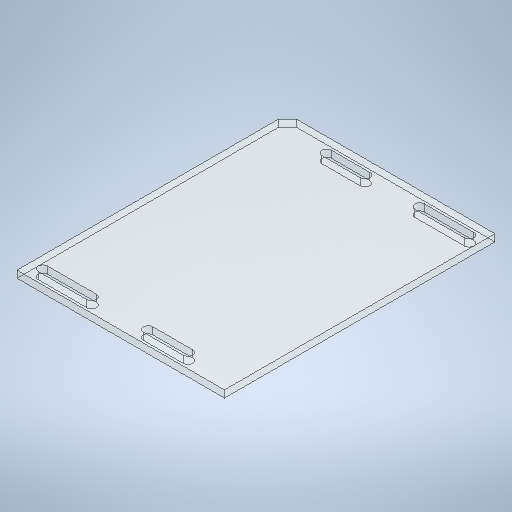
# Autodesk Inventor part: Flex Holder V1 TPMockup
Saved by Autodesk Inventor 2025 (Build 290162000, 162)
## iProperties
Created: 2025-07-01
Part Number: Flex Holder V1 TPMockup
Material: Thermoplastic Resin
Document SubType Name: Modeling
Designer: Caleb Fangmeier
Density: 1.28 g/cm^3
Appearance: Clear
Author: Caleb Fangmeier
Autodesk Inventor part; units mm, degrees
ref_plane "YZ Plane" through (0, 0, 0) normal (1, 0, 0) x (0, 1, 0)
ref_plane "XZ Plane" through (0, 0, 0) normal (0, 1, 0) x (-1, 0, 0)
ref_plane "XY Plane" through (0, 0, 0) normal (0, 0, 1) x (1, 0, 0)
sketch "Sketch1" plane through (0, 0, 0) normal (0, 1, 0) x (-1, 0, 0)
  line L0 (-22.05, -28.75) -> (22.05, -28.75)
  line L1 (22.05, -28.75) -> (22.05, 28.75)
  line L2 (22.05, 28.75) -> (-22.05, 28.75)
  line L3 (-22.05, 28.75) -> (-22.05, -28.75)
  line L4 (-22.05, -28.75) -> (22.05, 28.75) construction
  line L5 (22.05, -28.75) -> (-22.05, 28.75) construction
  point P0 (0, 0)
  dimension "d0" = 57.5
  dimension "d1" = 44.1
  constraints: 12 end point, 2 midpoint, 2 parallel, 1 horizontal, 1 perpendicular
  measures "d0" distance of L0.end L1.end
  measures "d1" distance of L1.end L2.end
extrude "Extrusion1" add sketch "Sketch1" along normal blind 1.5
sketch "Sketch4" plane through (0, 1.5, 0) normal (0, 1, 0) x (1, 0, 0)
  line L0 (22.6381, -25.9185) -> (13.7388, -25.9185)
  line L1 (13.7388, -25.9185) -> (13.7388, -21.956)
  line L2 (13.7388, -21.956) -> (22.6381, -21.956)
  line L3 (22.6381, -21.956) -> (22.6381, -25.9185)
  line L4 (11.4165, -21.956) -> (0.7633, -21.956)
  line L5 (0.7633, -21.956) -> (0.7633, -24.4569)
  line L6 (0.7633, -24.4569) -> (11.4165, -24.4569)
  line L7 (11.4165, -24.4569) -> (11.4165, -21.956)
  line L8 (-0.6658, -26.6006) -> (-6.707, -26.6006)
  line L9 (-6.707, -26.6006) -> (-6.707, -22.3783)
  line L10 (-6.707, -22.3783) -> (-0.6658, -22.3783)
  line L11 (-0.6658, -22.3783) -> (-0.6658, -26.6006)
  line L12 (-6.707, -24.392) -> (-14.5426, -24.392)
  line L13 (-14.5426, -24.392) -> (-14.5426, -21.0953)
  line L14 (-14.5426, -21.0953) -> (-6.707, -21.0953)
  line L15 (-6.707, -21.0953) -> (-6.707, -24.392)
  line L16 (-14.5426, -21.0953) -> (-11.8996, -21.0953)
  line L17 (-11.8996, -21.0953) -> (-11.8996, -19.5363)
  line L18 (-11.8996, -19.5363) -> (-14.5426, -19.5363)
  line L19 (-14.5426, -19.5363) -> (-14.5426, -21.0953)
  line L20 (-21.1238, -24.2621) -> (-17.4211, -24.2621)
  line L21 (-17.4211, -24.2621) -> (-17.4211, -21.956)
  line L22 (-17.4211, -21.956) -> (-21.1238, -21.956)
  line L23 (-21.1238, -21.956) -> (-21.1238, -24.2621)
  line L24 (5.6616, -20.7705) -> (1.894, -20.7705)
  line L25 (1.894, -20.7705) -> (1.894, -17.3277)
  line L26 (1.894, -17.3277) -> (5.6616, -17.3277)
  line L27 (5.6616, -17.3277) -> (5.6616, -20.7705)
  line L28 (-2.848, -19.9261) -> (-5.2515, -19.9261)
  line L29 (-5.2515, -19.9261) -> (-5.2515, -18.3346)
  line L30 (-5.2515, -18.3346) -> (-2.848, -18.3346)
  line L31 (-2.848, -18.3346) -> (-2.848, -19.9261)
  line L32 (-17.2689, -17.0029) -> (-14.5426, -17.0029)
  line L33 (-14.5426, -17.0029) -> (-14.5426, -13.4952)
  line L34 (-14.5426, -13.4952) -> (-17.2689, -13.4952)
  line L35 (-17.2689, -13.4952) -> (-17.2689, -17.0029)
  line L36 (15.925, -11.4814) -> (12.4173, -11.4814)
  line L37 (12.4173, -11.4814) -> (12.4173, -14.7294)
  line L38 (12.4173, -14.7294) -> (15.925, -14.7294)
  line L39 (15.925, -14.7294) -> (15.925, -11.4814)
  line L40 (-2.1335, 9.0455) -> (1.894, 9.0455)
  line L41 (1.894, 9.0455) -> (1.894, -8.9481)
  line L42 (1.894, -8.9481) -> (-2.1335, -8.9481)
  line L43 (-2.1335, -8.9481) -> (-2.1335, 9.0455)
  line L44 (4.5573, 3.3291) -> (1.6991, 3.3291)
  line L45 (1.6991, 3.3291) -> (1.6991, 0.6009)
  line L46 (1.6991, 0.6009) -> (4.5573, 0.6009)
  line L47 (4.5573, 0.6009) -> (4.5573, 3.3291)
  line L48 (-17.5287, 13.7631) -> (-14.1519, 13.7631)
  line L49 (-14.1519, 13.7631) -> (-14.1519, 10.4096)
  line L50 (-14.1519, 10.4096) -> (-17.5287, 10.4096)
  line L51 (-17.5287, 10.4096) -> (-17.5287, 13.7631)
  line L52 (16.8052, 16.3739) -> (14.7212, 16.3739)
  line L53 (14.7212, 16.3739) -> (14.7212, 12.9633)
  line L54 (14.7212, 12.9633) -> (16.8052, 12.9633)
  line L55 (16.8052, 12.9633) -> (16.8052, 16.3739)
  line L56 (-23.3919, 26.0219) -> (-13.2211, 26.0219)
  line L57 (-13.2211, 26.0219) -> (-13.2211, 21.0711)
  line L58 (-13.2211, 21.0711) -> (-23.3919, 21.0711)
  line L59 (-23.3919, 21.0711) -> (-23.3919, 26.0219)
  line L60 (-20.3793, 16.7032) -> (-17.8455, 16.7032)
  line L61 (-17.8455, 16.7032) -> (-17.8455, 19.4346)
  line L62 (-17.8455, 19.4346) -> (-20.3793, 19.4346)
  line L63 (-20.3793, 19.4346) -> (-20.3793, 16.7032)
  line L64 (-11.1745, 21.8169) -> (-0.7032, 21.8169)
  line L65 (-0.7032, 21.8169) -> (-0.7032, 24.5446)
  line L66 (-0.7032, 24.5446) -> (-11.1745, 24.5446)
  line L67 (-11.1745, 24.5446) -> (-11.1745, 21.8169)
  line L68 (-2.5673, 18.6812) -> (-4.8458, 18.6812)
  line L69 (-4.8458, 18.6812) -> (-4.8458, 22.2038)
  line L70 (-4.8458, 22.2038) -> (-2.5673, 22.2038)
  line L71 (-2.5673, 22.2038) -> (-2.5673, 18.6812)
  line L72 (0.9146, 27.1153) -> (6.539, 27.1153)
  line L73 (6.539, 27.1153) -> (6.539, 22.2038)
  line L74 (6.539, 22.2038) -> (0.9146, 22.2038)
  line L75 (0.9146, 22.2038) -> (0.9146, 27.1153)
  line L76 (2.2307, 17.9158) -> (4.5573, 17.9158)
  line L77 (4.5573, 17.9158) -> (4.5573, 22.2038)
  line L78 (4.5573, 22.2038) -> (2.2307, 22.2038)
  line L79 (2.2307, 22.2038) -> (2.2307, 17.9158)
  line L80 (6.0899, 24.1958) -> (14.5454, 24.1958)
  line L81 (14.5454, 24.1958) -> (14.5454, 21.5323)
  line L82 (14.5454, 21.5323) -> (6.0899, 21.5323)
  line L83 (6.0899, 21.5323) -> (6.0899, 24.1958)
  line L84 (14.2886, 21.5323) -> (11.9019, 21.5323)
  line L85 (11.9019, 21.5323) -> (11.9019, 19.3557)
  line L86 (11.9019, 19.3557) -> (14.2886, 19.3557)
  line L87 (14.2886, 19.3557) -> (14.2886, 21.5323)
  line L88 (21.4363, 24.0758) -> (17.64, 24.0758)
  line L89 (17.64, 24.0758) -> (17.64, 21.5323)
  line L90 (17.64, 21.5323) -> (21.4363, 21.5323)
  line L91 (21.4363, 21.5323) -> (21.4363, 24.0758)
  point P0 (0, 0)
  point P1 (6.539, 24.1958)
  point P2 (6.0899, 22.2038)
  constraints: 184 end point, 46 parallel, 23 perpendicular, 22 horizontal, 3 point on line
extrude "Clearance Cutouts" [suppressed]
sketch "Sketch5" plane through (0, 1.5, 0) normal (0, 1, 0) x (1, 0, 0)
  line L0 (19.55, 25.75) -> (9.039, 25.75) construction
  line L1 (19.55, 26.75) -> (9.039, 26.75)
  line L2 (9.039, 24.75) -> (19.55, 24.75)
  arc A0 (19.55, 24.75) -> (19.55, 26.75) centre (19.55, 25.75) ccw
  arc A1 (9.039, 26.75) -> (9.039, 24.75) centre (9.039, 25.75) ccw
  line L3 (22.05, -28.75) -> (22.05, 28.75) projected
  line L4 (-2.5854, 25.75) -> (-10.7211, 25.75) construction
  line L5 (-2.5854, 24.75) -> (-10.7211, 24.75)
  line L6 (-10.7211, 26.75) -> (-2.5854, 26.75)
  arc A2 (-2.5854, 24.75) -> (-2.5854, 26.75) centre (-2.5854, 25.75) ccw
  arc A3 (-10.7211, 26.75) -> (-10.7211, 24.75) centre (-10.7211, 25.75) ccw
  line L7 (-19.55, -25.75) -> (-9.207, -25.75) construction
  line L8 (-22.05, -28.75) -> (22.05, -28.75) projected
  line L9 (-19.55, -26.75) -> (-9.207, -26.75)
  line L10 (-9.207, -24.75) -> (-19.55, -24.75)
  arc A4 (-19.55, -24.75) -> (-19.55, -26.75) centre (-19.55, -25.75) ccw
  arc A5 (-9.207, -26.75) -> (-9.207, -24.75) centre (-9.207, -25.75) ccw
  line L11 (-22.05, 28.75) -> (-22.05, -28.75) projected
  line L12 (2.8342, -25.75) -> (11.2388, -25.75) construction
  line L13 (2.8342, -26.75) -> (11.2388, -26.75)
  line L14 (11.2388, -24.75) -> (2.8342, -24.75)
  arc A6 (2.8342, -24.75) -> (2.8342, -26.75) centre (2.8342, -25.75) ccw
  arc A7 (11.2388, -26.75) -> (11.2388, -24.75) centre (11.2388, -25.75) ccw
  line L15 (22.05, 28.75) -> (-22.05, 28.75) projected
  point P0 (0, 0)
  point P1 (14.2945, 25.75)
  point P2 (8.039, 25.75)
  point P3 (20.55, 25.75)
  point P4 (-6.6533, 25.75)
  point P5 (-1.5854, 25.75)
  point P6 (-11.7211, 25.75)
  point P7 (-14.3785, -25.75)
  point P8 (-8.207, -25.75)
  point P9 (-20.55, -25.75)
  point P10 (7.0365, -25.75)
  point P11 (1.8342, -25.75)
  point P12 (12.2388, -25.75)
  dimension "d23" = 2
  dimension "d26" = 1.5
  dimension "d30" = 1
  dimension "d31" = 1
  dimension "d34" = 1.5
  dimension "d35" = 1
  dimension "d44" = 3
  dimension "d45" = 15.3967
  dimension "d46" = 10.1357
  dimension "d47" = 3
  dimension "d48" = 12.511
  dimension "d49" = 3
  dimension "d50" = 3
  dimension "d51" = 10.4046
  dimension "d52" = 9.8112
  dimension "d53" = 12.343
  constraints: 32 end point, 24 point on circle, 16 tangent, 8 centre point, 5 parallel, 4 midpoint, 3 horizontal
  measures "d23" diameter of A1
  measures "d26" distance from line of L3 point (20.55, 25.75)
  measures "d30" radius of A2
  measures "d31" radius of A5
  measures "d34" distance from line of L11 point (-20.55, -25.75)
  measures "d35" radius of A7
  measures "d44" distance from line of L15 point (-6.653, 25.75)
  measures "d45" distance from line of L11 point (-6.653, 25.75)
  measures "d46" distance of point (-1.585, 25.75) point (-11.721, 25.75)
  measures "d47" distance from line of L15 point (14.294, 25.75)
  measures "d48" distance of point (20.55, 25.75) point (8.039, 25.75)
  measures "d49" distance from line of L8 point (-14.378, -25.75)
  measures "d50" distance from line of L8 point (7.036, -25.75)
  measures "d51" distance of point (1.834, -25.75) point (12.239, -25.75)
  measures "d52" distance from line of L3 point (12.239, -25.75)
  measures "d53" distance of point (-20.55, -25.75) point (-8.207, -25.75)
extrude "Extrusion4" cut sketch "Sketch5" against normal blind 1.5 contours A0 L2 A1 L1 | L5 A3 L6 A2 | A4 L10 A5 L9 | A6 L14 A7 L13
chamfer "Chamfer1" distance 2 angle 45 1 edges at (-22.05, 0.75, -28.75)
body "Solid1"
